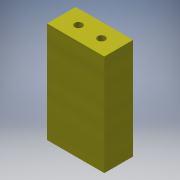
# Autodesk Inventor part: Garalite Support
Saved by Autodesk Inventor 2017 (Build 210142000, 142)
## iProperties
Created: 2017-03-02
Part Number: Garalite Support
Material: Generic
Document SubType Name: Modeling
Designer: coffmant
Density: 1 g/cm^3
Appearance: Canary
Quantity: 1
Author: coffmant
Autodesk Inventor part; units mm, degrees
ref_plane "YZ Plane" through (0, 0, 0) normal (1, 0, 0) x (0, 1, 0)
ref_plane "XZ Plane" through (0, 0, 0) normal (0, 1, 0) x (-1, 0, 0)
ref_plane "XY Plane" through (0, 0, 0) normal (0, 0, 1) x (1, 0, 0)
sketch "Sketch1" plane through (0, 0, 0) normal (0, 1, 0) x (-1, 0, 0)
  line L0 (0, 0) -> (-31.75, 0)
  line L1 (-31.75, 0) -> (-31.75, -15.875)
  line L2 (-31.75, -15.875) -> (0, -15.875)
  line L3 (0, -15.875) -> (0, 0)
  dimension "d0" = 15.875
  dimension "d1" = 31.75
  constraints: 8 end point, 2 parallel, 1 horizontal, 1 perpendicular
  measures "d0" distance between parallel lines of L2 L0
  measures "d1" distance between parallel lines of L3 L1
extrude "Extrusion1" add sketch "Sketch1" along normal blind 55.88
sketch "Sketch2" plane through (0, 55.88, 0) normal (0, 1, 0) x (1, 0, 0)
  line L0 (0, 15.875) -> (0, 0) projected
  line L1 (31.75, 0) -> (31.75, 15.875) projected
  line L2 (31.75, 15.875) -> (0, 15.875) projected
  line L3 (0, 0) -> (31.75, 0) projected
  point P0 (9.525, 7.9375)
  point P1 (22.225, 7.9375)
  dimension "d5" = 12.7
  dimension "d25" = 15.875
  dimension "d26" = 7.9375
  dimension "d27" = 9.525
  constraints: 1 horizontal alignment
  measures "d5" distance of point (9.525, 7.938) point (22.225, 7.938)
  measures "d25" distance between parallel lines of L2 L3
  measures "d26" distance from line of point (9.525, 7.938) L3
  measures "d27" distance from line of L0 point (9.525, 7.938)
hole "Hole1" at (9.525, 55.88, -7.9375) at (22.225, 55.88, -7.9375) direction (0, -1, 0) diameter 4.2164 depth 6.35 tip angle 118
sketch "Sketch3" plane through (0, 0, 0) normal (0, -1, 0) x (1, 0, 0)
  circle A0 centre (9.525, -7.9375) radius 2.1082 projected
  circle A1 centre (22.225, -7.9375) radius 2.1082 projected
  point P0 (0, 0)
  constraints: 2 coincident
hole "Hole2" at (9.525, 0, -7.9375) at (22.225, 0, -7.9375) direction (0, 1, 0) diameter 4.2164 depth 6.35 tip angle 118
equation "\"d26\" = 0.5 * d25"
body "Solid1"
